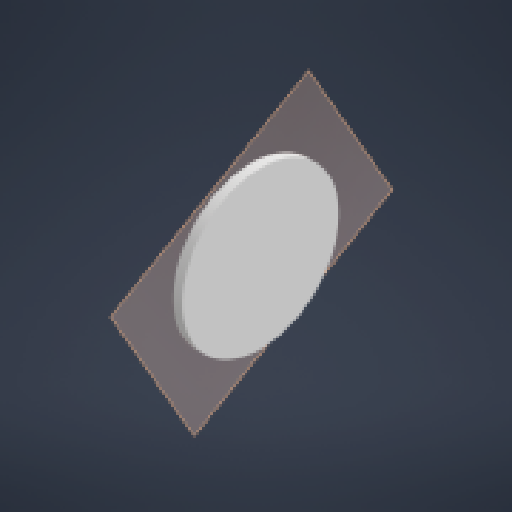
# Autodesk Inventor part: Ball Bearing Spacer
Saved by Autodesk Inventor 2023 (Build 270158000, 158)
## iProperties
Created: 2022-10-05
Part Number: Ball Bearing Spacer
Material: Generic
Document SubType Name: Modeling
Designer: izack
Density: 1 g/cm^3
Appearance: Default
Author: izack
Autodesk Inventor part; units mm, degrees
ref_plane "YZ Plane" through (0, 0, 0) normal (1, 0, 0) x (0, 1, 0)
ref_plane "XZ Plane" through (0, 0, 0) normal (0, 1, 0) x (-1, 0, 0)
ref_plane "XY Plane" through (0, 0, 0) normal (0, 0, 1) x (1, 0, 0)
ref_plane "Work Plane1" through (-5.75, 1.53, 2.65) normal (1, 0, 0) x (0, -0.8660254, -0.5)
sketch "Sketch1" plane through (-5.75, 1.53, 2.65) normal (1, 0, 0) x (0, -0.8660254, -0.5)
  circle A0 centre (1.3017, 5.7033) radius 2.1213
  circle A1 centre (1.3017, 5.7033) radius 2.4213
  circle A2 centre (-3.6474, 4.5737) radius 2.4213
  circle A3 centre (-5.85, 0) radius 2.4213
  circle A4 centre (-3.6474, -4.5737) radius 2.4213
  circle A5 centre (1.3017, -5.7033) radius 2.4213
  circle A6 centre (5.2707, -2.5382) radius 2.4213
  circle A7 centre (5.2707, 2.5382) radius 2.4213
  circle A8 centre (0, 0) radius 8.5
  circle A9 centre (0, 0) radius 3.1
  point P0 (2.65, 1.53)
  point P1 (7.4522, -3.5888)
  point P2 (7.4522, 3.5888)
  point P3 (1.8405, -8.0639)
  point P4 (-5.1571, -6.4668)
  point P5 (-8.2713, 0)
  point P6 (-5.1571, 6.4668)
  point P7 (1.8405, 8.0639)
  dimension "d0" = 0.3
  dimension "d3" = 360
  dimension "d7" = 17
  dimension "d9" = 6.2
  constraints: 10 centre point, 2 coincident, 17 other
  measures "d0" radial gap between concentric circles of A0 A1
  measures "d7" diameter of A8
  measures "d9" diameter of A9
extrude "Extrusion1" add sketch "Sketch1" along normal blind 1 contours A8
ref_plane "Work Plane2" through (-5, 1.53, 2.65) normal (1, 0, 0) x (0, -0.8660254, -0.5)
sketch "Sketch2" plane through (-5, 1.53, 2.65) normal (1, 0, 0) x (0, -0.8660254, -0.5)
  circle A0 centre (5.2707, 2.5382) radius 2.25
  circle A1 centre (5.2707, 2.5382) radius 2.55
  line L0 (5.2707, 5.0882) -> (5.2707, -0.0118)
  point P0 (2.65, 1.53)
  dimension "d10" = 0.3
  constraints: 2 centre point, 2 end point, 2 point on circle, 2 other
  measures "d10" radial gap between concentric circles of A0 A1
revolve "Revolution1" cut sketch "Sketch2" angle 360 about axis through (-5, -0.4904, -4.3919) along (0, -0.5, 0.8660254) picked at (6.024, 2.987) picked at (7.6994, 2.3491) contours A0 L0 | A0 L0 A1
pattern_circular "Circular Pattern1" count 7 over 360 about axis through (-5.75, 1.53, 2.65) along (1, 0, 0) of "Revolution1"
body "Solid1"
